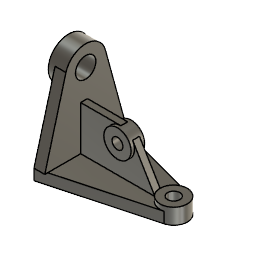
MaRS_Q5_f (Autodesk Fusion 360 design; units mm, degrees)
part number: 2026-05-30-18-56-35-103
Autodesk Fusion 360 part; units mm, degrees
sketch "Sketch1" plane through (0, 0, 0) normal (0, 0, 1) x (1, 0, 0)
  line L0 (0.1058, -52.6202) -> (0.1058, 67.3798)
  line L1 (0.1058, 67.3798) -> (0.1058, 7.3798)
  circle A0 centre (145.1058, 7.3798) radius 9
  circle A1 centre (145.1058, 7.3798) radius 20
  line L2 (0.1058, 67.3798) -> (150.3351, 26.684)
  line L3 (0.1058, -52.6202) -> (150.3351, -11.9245)
  dimension "d1" = 120
  dimension "d2" = 60
  dimension "d3" = 145
  dimension "d4" = 18
  dimension "d5" = 40
  constraint vertical L0
  constraint parallel L0 L1
  constraint concentric A0 A1
  constraint coincident A1 L2.end
  constraint tangent A1 L2
  constraint coincident A1 L3.end
  constraint tangent A1 L3
  measures "d1" distance of L0.start L0.end
  measures "d2" distance of L0.end L1.end
  measures "d3" distance of L1.end A0.centre
  measures "d4" diameter of A0
  measures "d5" diameter of A1
extrude "Extrude1" add sketch "Sketch1" along normal blind 16 contours L0 L1 A1 L2 L3
extrude "Extrude2" add sketch "Sketch1" along normal blind 23 contours A1
sketch "Sketch2" plane through (0, 0, 16) normal (0, 0, 1) x (-1, 0, 0)
  line L0 (-0.1058, -67.3798) -> (-0.1058, 52.6202)
  line L1 (-0.1058, 52.6202) -> (-150.3351, 11.9245)
  arc A0 (-150.3351, -26.684) -> (-150.3351, 11.9245) centre (-145.1058, -7.3798) ccw
  line L2 (-150.3351, -26.684) -> (-0.1058, -67.3798)
sketch "Sketch3" plane through (0, 0, 0) normal (1, 0, 0) x (0, 1, 0)
sketch "Sketch4" plane through (0, 0, 0) normal (1, 0, 0) x (0, 1, 0)
  line L0 (-52.6, 16) -> (67.3803, 16)
  line L1 (67.3803, 16) -> (7.3902, 16)
  line L2 (7.3902, 16) -> (7.3902, 122)
  circle A0 centre (7.3902, 122) radius 30
  circle A1 centre (7.3902, 122) radius 15
  line L3 (-52.6, 16) -> (-21.5537, 129.8901)
  line L4 (67.3803, 16) -> (36.334, 129.8901)
  dimension "d10" = 106
  dimension "d11" = 60
  dimension "d12" = 30
  constraint horizontal L0
  constraint midpoint L0 L1.end
  constraint perpendicular L0 L2
  constraint coincident L2.end A0.centre
  constraint concentric A0 A1
  constraint coincident A0 L3.end
  constraint tangent A0 L3
  constraint coincident A0 L4.end
  constraint tangent A0 L4
  measures "d10" distance of L1.end L2.end
  measures "d11" diameter of A0
  measures "d12" diameter of A1
extrude "Extrude3" add sketch "Sketch4" along normal blind 16 contours L0 L2 A0 L3 | L0 L1 L2 A0 L4
sketch "Sketch5" plane through (16, 0, 0) normal (1, 0, 0) x (0, 1, 0)
  line L0 (-52.6, 16) -> (-48.3146, 16)
  line L1 (-48.3146, 16) -> (63.0742, 16)
  line L2 (63.0742, 16) -> (67.3803, 16)
  line L3 (67.3803, 16) -> (36.334, 129.8901)
  arc A0 (-21.5537, 129.8901) -> (36.334, 129.8901) centre (7.3902, 122) ccw
  line L4 (-21.5537, 129.8901) -> (-52.6, 16)
  circle A1 centre (7.3902, 122) radius 15
  circle A2 centre (7.3902, 122) radius 30
  dimension "d15" = 30
  dimension "d16" = 60
  constraint concentric A0 A1
  constraint concentric A1 A2
  measures "d15" diameter of A1
  measures "d16" diameter of A2
extrude "Extrude4" add sketch "Sketch5" against normal blind 25 contours A0 A2
sketch "Sketch6" plane through (0, 0, 0) normal (0, 1, 0) x (1, 0, 0)
  line L0 (0, 0) -> (0, -61)
  circle A0 centre (75, -61) radius 20
  circle A1 centre (75, -61) radius 8
  line L1 (75, -81) -> (16, -81)
  line L2 (124.9247, -16.1323) -> (92.1937, -71.2165)
  line L3 (16, -81) -> (16, -16)
  line L4 (16, -16) -> (124.9247, -16.1323)
  dimension "d19" = 61
  dimension "d20" = 75
  dimension "d21" = 40
  dimension "d22" = 16
  constraint coincident L0.start origin
  constraint vertical L0
  constraint concentric A0 A1
  constraint coincident A0 L1.start
  constraint horizontal L1
  constraint coincident A0 L2.end
  constraint tangent A0 L2
  constraint perpendicular L1 L3
  measures "d19" distance of L0.start L0.end
  measures "d20" distance of L0.end A0.centre
  measures "d21" diameter of A0
  measures "d22" diameter of A1
sketch "Sketch7" plane through (16, 0, 0) normal (1, 0, 0) x (0, 1, 0)
  circle A0 centre (7.3902, 122) radius 15
  line L0 (-52.6, 16) -> (-48.3146, 16)
  line L1 (-48.3146, 16) -> (63.0742, 16)
  line L2 (63.0742, 16) -> (67.3803, 16)
  line L3 (67.3803, 16) -> (36.334, 129.8901)
  arc A1 (36.334, 129.8901) -> (-21.5537, 129.8901) centre (7.3902, 122) ccw
  line L4 (-21.5537, 129.8901) -> (-52.6, 16)
sketch "Sketch8" plane through (0, 0, 0) normal (0, 1, 0) x (1, 0, 0)
extrude "Extrude5" add sketch "Sketch6" along normal blind 10 contours A0 L1 L2 L3 L4
extrude "Extrude6" add sketch "Sketch6" along normal blind 15 contours A0
extrude "Extrude7" add sketch "Sketch6" against normal blind 5 contours A0
